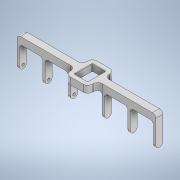
# Autodesk Inventor part: y arm connection
Saved by Autodesk Inventor 2021 (Build 250183000, 183)
## iProperties
Created: 2021-06-24
Part Number: y arm connection
Material: Generic
Document SubType Name: Modeling
Designer: josep
Density: 1 g/cm^3
Appearance: Default
Author: josep
Autodesk Inventor part; units mm, degrees
ref_plane "YZ Plane" through (0, 0, 0) normal (1, 0, 0) x (0, 1, 0)
ref_plane "XZ Plane" through (0, 0, 0) normal (0, 1, 0) x (-1, 0, 0)
ref_plane "XY Plane" through (0, 0, 0) normal (0, 0, 1) x (1, 0, 0)
sketch "Sketch1" plane through (0, 0, 0) normal (1, 0, 0) x (0, 1, 0)
  line L0 (0, 0) -> (0, -19)
  line L1 (0, 0) -> (0, 19)
  line L2 (0, 19) -> (-50, 19)
  line L3 (-50, 19) -> (-50, 29)
  line L4 (-50, 29) -> (0, 29)
  line L5 (0, 29) -> (0, 19)
  line L6 (0, -19) -> (-50, -19)
  line L7 (-50, -19) -> (-50, -29)
  line L8 (-50, -29) -> (0, -29)
  line L9 (0, -29) -> (0, -19)
  dimension "d0" = 19
  dimension "d1" = 19
  dimension "d2" = 50
  dimension "d3" = 10
  dimension "d4" = 50
  dimension "d5" = 10
  constraints: 20 end point, 4 perpendicular, 2 horizontal, 2 parallel, 2 vertical
  measures "d0" distance of L0.start L0.end
  measures "d1" distance of L0.start L1.end
  measures "d2" distance of L1.end L2.end
  measures "d3" distance of L2.end L3.end
  measures "d4" distance of L8.end L7.end
  measures "d5" distance of L7.end L6.end
extrude "Extrusion1" add sketch "Sketch1" along normal blind 347
sketch "Sketch2" plane through (0, 0, -19) normal (0, 1, 0) x (1, 0, 0)
  line L0 (-41.2158, -120.6879) -> (285.948, -120.6879)
  line L1 (285.948, -120.6879) -> (285.948, 128.9897)
  line L2 (285.948, 128.9897) -> (-41.2158, 128.9897)
  line L3 (-41.2158, 128.9897) -> (-41.2158, -120.6879)
  line L4 (-65.3226, -208.5055) -> (414.2306, -208.5055)
  line L5 (414.2306, -208.5055) -> (414.2306, 175.4814)
  line L6 (414.2306, 175.4814) -> (-65.3226, 175.4814)
  line L7 (-65.3226, 175.4814) -> (-65.3226, -208.5055)
  point P0 (0, -19)
  constraints: 16 end point, 4 parallel, 2 horizontal, 2 perpendicular
extrude "Extrusion2" cut sketch "Sketch2" against normal blind 25 contours L3 L2 L1 L0 | L7 L6 L5 L4
sketch "Sketch3" plane through (347, 0, 0) normal (1, 0, 0) x (0, 0, -1)
  line L0 (-29, -25) -> (-29, -50) projected
  line L1 (-29, -38.3566) -> (-26.5, -38.3566)
  line L2 (-26.5, -38.3566) -> (-25.5, -38.3566)
  line L3 (-29, -25) -> (-19, -25) projected
  line L4 (-25.5, -25) -> (-25.5, -50)
  line L5 (-29, -50) -> (-19, -50) projected
  line L6 (-29, -25) -> (-25.5, -25)
  line L7 (-25.5, -25) -> (-25.5, -50)
  line L8 (-25.5, -50) -> (-29, -50)
  line L9 (-29, -50) -> (-29, -25)
  line L10 (19, -50) -> (29, -50) projected
  line L11 (29, -25) -> (25.5, -25)
  line L12 (25.5, -25) -> (25.5, -50)
  line L13 (25.5, -50) -> (29, -50)
  line L14 (29, -50) -> (29, -25)
  point P0 (0, 0)
  dimension "d10" = 2.5
  dimension "d11" = 1
  dimension "d12" = 3.5
  constraints: 22 end point, 5 point on line, 4 parallel, 3 horizontal, 2 perpendicular, 1 vertical
  measures "d10" distance of L1.start L1.end
  measures "d11" distance of L1.end L2.end
  measures "d12" distance of L13.end L12.end
extrude "Extrusion3" cut sketch "Sketch3" against normal blind 373
sketch "Sketch4" plane through (0, -25, -19) normal (0, 1, 0) x (1, 0, 0)
  line L0 (0, -38) -> (347, -38) projected
  line L1 (277.7024, -38) -> (249.7024, -38)
  line L2 (249.7024, -38) -> (249.7024, 0)
  line L3 (347, 0) -> (0, 0) projected
  line L4 (277.7024, -38) -> (277.7024, 0)
  line L5 (277.7024, 0) -> (287.7024, 0)
  line L6 (287.7024, -36.5) -> (287.7024, -38)
  line L7 (229.7024, -11.5) -> (205.0573, -11.5)
  line L8 (297.7024, -11.5) -> (336.2476, -11.5)
  line L9 (336.2476, -11.5) -> (336.2476, -26.5)
  line L10 (336.2476, -26.5) -> (297.7024, -26.5)
  arc A0 (297.7024, -26.5) -> (287.7024, -36.5) centre (297.7024, -36.5) ccw
  line L11 (287.7024, 0) -> (287.7024, -1.5)
  arc A1 (287.7024, -1.5) -> (297.7024, -11.5) centre (297.7024, -1.5) ccw
  line L12 (287.7024, -38) -> (277.7024, -38)
  line L13 (249.7024, 0) -> (239.7024, 0)
  line L14 (239.7024, 0) -> (239.7024, -1.5)
  line L15 (239.7024, -36.5) -> (239.7024, -38)
  line L16 (229.7024, -26.5) -> (205.0573, -26.5)
  line L17 (205.0573, -26.5) -> (205.0573, -11.5)
  arc A2 (229.7024, -11.5) -> (239.7024, -1.5) centre (229.7024, -1.5) ccw
  arc A3 (239.7024, -36.5) -> (229.7024, -26.5) centre (229.7024, -36.5) ccw
  line L18 (249.7024, -38) -> (239.7024, -38)
  point P0 (0, -19)
  point P1 (239.7024, -19)
  point P2 (334.5589, -26.5)
  dimension "d15" = 28
  dimension "d16" = 10
  dimension "d19" = 15
  dimension "d20" = 10
  dimension "d21" = 10
  dimension "d22" = 10
  dimension "d23" = 10
  constraints: 34 end point, 17 point on line, 8 perpendicular, 8 point on circle, 8 tangent, 4 centre point, 2 collinear, 1 equal radius
  measures "d15" distance of L1.start L1.end
  measures "d16" distance of L4.end L5.end
  measures "d19" distance of L8.end L9.end
  measures "d20" radius of A0
  measures "d21" radius of A1
  measures "d22" distance of L2.end L13.end
  measures "d23" radius of A2
extrude "Extrusion4" add sketch "Sketch4" against normal blind 25 contours L15 A3 L16 L17 L7 A2 L14 L3 L2 L0 | L4 L3 L11 A1 L8 L9 L10 A0 L6 L0
sketch "Sketch5" plane through (0, -25, -19) normal (0, 1, 0) x (1, 0, 0)
  line L0 (249.7024, -38) -> (277.7024, -38) projected
  line L1 (277.7024, -38) -> (277.7024, -48)
  line L2 (277.7024, -48) -> (249.7024, -48)
  line L3 (347, -44.5) -> (0, -44.5) projected
  line L4 (287.7024, -38) -> (347, -38) projected
  line L5 (287.7024, -38) -> (287.7024, 0)
  arc A0 (277.7024, -48) -> (287.7024, -38) centre (277.7024, -38) ccw
  arc A1 (239.7024, -36.5) -> (229.7024, -26.5) centre (229.7024, -36.5) ccw projected
  line L6 (239.7024, 0) -> (239.7024, -38)
  arc A2 (239.7024, -38) -> (249.7024, -48) centre (249.7024, -38) ccw
  line L7 (249.7024, 0) -> (277.7024, 0) projected
  line L8 (277.7024, 0) -> (277.7024, 10)
  line L9 (277.7024, 10) -> (249.7024, 10)
  arc A3 (287.7024, 0) -> (277.7024, 10) centre (277.7024, 0) ccw
  arc A4 (249.7024, 10) -> (239.7024, 0) centre (249.7024, 0) ccw
  line L10 (277.7024, -38) -> (249.7024, -38)
  line L11 (249.7024, -38) -> (249.7024, 0)
  line L12 (249.7024, 0) -> (277.7024, 0)
  line L13 (277.7024, 0) -> (277.7024, -38)
  point P0 (0, -19)
  dimension "d26" = 10
  dimension "d27" = 10
  dimension "d28" = 10
  dimension "d29" = 10
  dimension "d30" = 10
  constraints: 20 end point, 9 tangent, 8 point on circle, 4 centre point, 4 point on line, 3 parallel, 3 perpendicular, 3 vertical, 1 equal radius, 1 horizontal
  measures "d26" distance of L0.end L1.end
  measures "d27" radius of A0
  measures "d28" radius of A2
  measures "d29" distance of L7.end L8.end
  measures "d30" radius of A3
extrude "Extrusion5" add sketch "Sketch5" against normal blind 25 contours L0 L1 L3 A2 L6 A4 L9 L8 L7 L11 | L13 L8 A3 L5 A0 L3 L1 | L3 A0 L1 | L1 L2 A2 L3
sketch "Sketch6" plane through (0, -25, -19) normal (0, 1, 0) x (1, 0, 0)
  arc A0 (287.7024, -1.5) -> (297.7024, -11.5) centre (297.7024, -1.5) ccw projected
  arc A1 (297.7024, -26.5) -> (287.7024, -36.5) centre (297.7024, -36.5) ccw projected
  line L0 (277.7024, -48) -> (249.7024, -48) projected
  line L1 (249.7024, -48) -> (277.7024, -48)
  arc A2 (277.7024, -48) -> (287.7024, -38) centre (277.7024, -38) ccw
  line L2 (249.7024, 10) -> (277.7024, 10) projected
  line L3 (277.7024, 10) -> (249.7024, 10)
  line L4 (239.7024, -36.5) -> (239.7024, -38) projected
  arc A3 (287.7024, 0) -> (277.7024, 10) centre (277.7024, 0) ccw
  arc A4 (249.7024, 10) -> (239.7024, 0) centre (249.7024, 0) ccw
  arc A5 (239.7024, -38) -> (249.7024, -48) centre (249.7024, -38) ccw
  line L5 (395.5953, -66.3707) -> (-113.6205, -66.3707)
  line L6 (-113.6205, -66.3707) -> (-113.6205, 72.1294)
  line L7 (-113.6205, 72.1294) -> (395.5953, 72.1294)
  line L8 (395.5953, 72.1294) -> (395.5953, -66.3707)
  line L9 (287.7024, -38) -> (349.7072, -27.7131)
  line L10 (349.7072, -27.7131) -> (348.1864, -4.5628)
  line L11 (348.1864, -4.5628) -> (318.7048, -5.5764)
  line L12 (318.7048, -5.5764) -> (293.2276, -4.5628)
  line L13 (347, 0) -> (287.7024, 0) projected
  line L14 (287.7024, 0) -> (293.2276, -4.5628)
  line L15 (0, -38) -> (239.7024, -38) projected
  line L16 (239.7024, -38) -> (183.3233, -27.7131)
  line L17 (183.3233, -27.7131) -> (188.9622, -13.5346)
  line L18 (239.7024, 0) -> (239.7024, -1.5) projected
  line L19 (188.9622, -13.5346) -> (239.7024, 0)
  point P0 (0, -19)
  point P1 (256.6196, -48)
  point P2 (272.9773, -48)
  point P3 (272.9773, 10)
  point P4 (258.3118, 10)
  dimension "d33" = 10
  dimension "d34" = 10
  constraints: 28 end point, 8 point on circle, 8 point on line, 4 centre point, 4 tangent, 2 equal radius, 2 parallel, 1 horizontal, 1 perpendicular
  measures "d33" radius of A2
  measures "d34" radius of A3
extrude "Extrusion6" cut sketch "Sketch6" against normal blind 113.5
sketch "Sketch7" plane through (336.2476, -25, 7.5) normal (1, 0, 0) x (0, 0, -1)
  line L0 (26.5, -25) -> (-11.5, -25) projected
  line L1 (15, 0) -> (15, -25) projected
  line L2 (-0.0488, -25) -> (15, -25)
  line L3 (15, -25) -> (15, 0)
  line L4 (15, 0) -> (-0.0488, 0)
  line L5 (-0.0488, 0) -> (-0.0488, -25)
  point P0 (7.5, 25)
  constraints: 8 end point, 2 parallel, 1 horizontal, 1 perpendicular, 1 point on line
extrude "Extrusion7" add sketch "Sketch7" along normal blind 320
sketch "Sketch8" plane through (205.0573, -50, 7.5) normal (0, -1, 0) x (1, 0, 0)
  arc A0 (34.6451, -25) -> (24.6451, -15) centre (24.6451, -25) ccw projected
  line L0 (24.6451, 0) -> (0, 0) projected
  line L1 (24.6451, -15) -> (19.6451, -15)
  line L2 (19.6451, -15) -> (19.6451, 0)
  line L3 (19.6451, 0) -> (24.6451, 0)
  line L4 (24.6451, 0) -> (24.6451, -15)
  point P0 (-205.0573, -7.5)
  dimension "d39" = 5
  constraints: 8 end point, 2 parallel, 1 horizontal, 1 perpendicular, 1 point on line
  measures "d39" distance of L2.end L3.end
extrude "Extrusion8" add sketch "Sketch8" along normal blind 50
sketch "Sketch9" plane through (224.7024, -50, -7.5) normal (-1, 0, 0) x (0, 0, 1)
  line L0 (0, -50) -> (15, -50) projected
  line L1 (7.5, -50) -> (7.5, -42.5)
  circle A0 centre (7.5, -42.5) radius 7.5
  line L2 (0, 0) -> (0, -50) projected
  line L3 (0, -42.5) -> (15, -42.5)
  line L4 (15, -42.5) -> (15, -50)
  line L5 (15, -50) -> (0, -50)
  line L6 (0, -50) -> (0, -42.5)
  point P0 (7.5, 50)
  point P1 (15, -42.5)
  dimension "d42" = 7.5
  constraints: 10 end point, 2 parallel, 2 point on circle, 1 centre point, 1 coincident, 1 horizontal, 1 midpoint, 1 perpendicular, 1 point on line, 1 vertical
  measures "d42" distance of L1.start L1.end
extrude "Extrusion9" cut sketch "Sketch9" against normal blind 50 contours L2 A0 L0 | A0 L4 L0
sketch "Sketch10" plane through (205.0573, -25, -7.5) normal (-1, 0, 0) x (0, 0, 1)
  line L0 (0, 0) -> (0, -25) projected
  line L1 (15, -25) -> (0, -25) projected
  line L2 (0, 0) -> (15, 0)
  line L3 (15, 0) -> (15, -25)
  line L4 (15, -25) -> (0, -25)
  line L5 (0, -25) -> (0, 0)
  point P0 (7.5, 25)
  constraints: 8 end point, 2 parallel, 1 horizontal, 1 perpendicular
extrude "Extrusion10" add sketch "Sketch10" along normal blind 318.75
sketch "Sketch11" plane through (224.7024, -50, -7.5) normal (0, -1, 0) x (1, 0, 0)
  line L0 (0, 0) -> (0, 15) projected
  line L1 (0, 7.5) -> (-50, 7.5)
  line L2 (0, 0) -> (-338.3951, 0) projected
  line L3 (0, 15) -> (-338.3951, 15) projected
  line L4 (-50, 0) -> (-55, 0)
  line L5 (-55, 0) -> (-55, 15)
  line L6 (-55, 15) -> (-50, 15)
  line L7 (-50, 15) -> (-50, 0)
  line L8 (-55, 7.5) -> (-105, 7.5)
  line L9 (-105, 0) -> (-110, 0)
  line L10 (-110, 0) -> (-110, 15)
  line L11 (-110, 15) -> (-105, 15)
  line L12 (-105, 15) -> (-105, 0)
  point P0 (-224.7024, 7.5)
  point P1 (-55, 0)
  point P2 (-110, 0)
  dimension "d47" = 50
  dimension "d48" = 5
  dimension "d49" = 50
  dimension "d50" = 5
  constraints: 20 end point, 4 horizontal, 4 parallel, 4 point on line, 2 midpoint, 2 perpendicular
  measures "d47" distance of L1.start L1.end
  measures "d48" distance of L5.end L6.end
  measures "d49" distance of L8.start L8.end
  measures "d50" distance of L10.end L11.end
extrude "Extrusion11" add sketch "Sketch11" along normal blind 50 contours L2 L5 L3 L7 | L2 L10 L3 L12
sketch "Sketch12" plane through (-113.6927, -50, -7.5) normal (0, -1, 0) x (1, 0, 0)
  line L0 (228.3951, 15) -> (228.3951, 0) projected
  line L1 (228.3951, 15) -> (-4838.5654, 15)
  line L2 (-4838.5654, 15) -> (-4838.5654, -3335.2499)
  line L3 (-4838.5654, -3335.2499) -> (228.3951, -3335.2499)
  line L4 (228.3951, -3335.2499) -> (228.3951, 15)
  point P0 (113.6927, 7.5)
  constraints: 8 end point, 2 parallel, 1 horizontal, 1 perpendicular
extrude "Extrusion12" cut sketch "Sketch12" against normal blind 50
sketch "Sketch13" plane through (114.7024, -100, -7.5) normal (-1, 0, 0) x (0, 0, 1)
  line L0 (15, 0) -> (0, 0) projected
  line L1 (7.5, 0) -> (7.5, 7.5)
  circle A0 centre (7.5, 7.5) radius 7.5
  line L2 (0, 50) -> (0, 7.5) projected
  line L3 (0, 7.5) -> (15, 7.5)
  line L4 (15, 7.5) -> (15, 0)
  line L5 (15, 0) -> (0, 0)
  line L6 (0, 0) -> (0, 7.5)
  point P0 (7.5, 100)
  point P1 (15, 7.5)
  dimension "d55" = 7.5
  constraints: 10 end point, 2 parallel, 1 centre point, 1 coincident, 1 horizontal, 1 midpoint, 1 perpendicular, 1 point on circle, 1 vertical
  measures "d55" distance of L1.start L1.end
sketch "Sketch14" plane through (277.7024, -25, -19) normal (-1, 0, 0) x (0, 0, 1)
  line L0 (38, -25) -> (0, -25) projected
  line L1 (38, 0) -> (0, 0)
  line L2 (0, 0) -> (0, -25)
  line L3 (0, -25) -> (38, -25)
  line L4 (38, -25) -> (38, 0)
  point P0 (19, 25)
  constraints: 8 end point, 2 parallel, 1 horizontal, 1 perpendicular
extrude "Extrusion13" add sketch "Sketch14" along normal blind 14
extrude "Extrusion14" cut sketch "Sketch13" against normal blind 183 contours L0 A0 L4 | L0 L6 A0
sketch "Sketch15" plane through (229.7024, -50, 7.5) normal (1, 0, 0) x (0, 0, -1)
  arc A0 (0, -42.5) -> (15, -42.5) centre (7.5, -42.5) ccw projected
  circle A1 centre (7.5, -42.5) radius 2.925
  point P0 (7.5, 50)
  dimension "d60" = 5.85
  constraints: 1 centre point, 1 coincident
  measures "d60" diameter of A1
extrude "Extrusion15" cut sketch "Sketch15" against normal blind 3.5
sketch "Sketch16" plane through (174.7024, -50, 7.5) normal (1, 0, 0) x (0, 0, -1)
  circle A0 centre (7.5, -42.5) radius 2.925
  point P0 (7.5, 50)
  dimension "d63" = 5.85
  constraints: 1 centre point
  measures "d63" diameter of A0
extrude "Extrusion16" cut sketch "Sketch16" against normal blind 3.5
sketch "Sketch17" plane through (119.7024, -50, 7.5) normal (1, 0, 0) x (0, 0, -1)
  arc A0 (0, -42.5) -> (15, -42.5) centre (7.5, -42.5) ccw projected
  circle A1 centre (7.5, -42.5) radius 2.925
  point P0 (7.5, 50)
  dimension "d66" = 5.85
  constraints: 1 centre point, 1 coincident
  measures "d66" diameter of A1
extrude "Extrusion17" cut sketch "Sketch17" against normal blind 3.5
sketch "Sketch18" plane through (263.7024, -25, -19) normal (-1, 0, 0) x (0, 0, 1)
  line L0 (-90.6404, 73.0269) -> (201.3127, 73.0269)
  line L1 (201.3127, 73.0269) -> (201.3127, -129.1917)
  line L2 (201.3127, -129.1917) -> (-90.6404, -129.1917)
  line L3 (-90.6404, -129.1917) -> (-90.6404, 73.0269)
  point P0 (19, 25)
  constraints: 8 end point, 2 parallel, 1 horizontal, 1 perpendicular
extrude "Extrusion18" cut sketch "Sketch18" against normal blind 599
mirror "Mirror1" about plane through (263.7024, -53.0824, 36.3362) normal (1, 0, 0)
sketch "Sketch19" plane through (0, -25, -19) normal (0, 1, 0) x (1, 0, 0)
  line L0 (36.6559, 37.945) -> (601.2573, 37.945)
  line L1 (601.2573, 37.945) -> (601.2573, -148.0607)
  line L2 (601.2573, -148.0607) -> (36.6559, -148.0607)
  line L3 (36.6559, -148.0607) -> (36.6559, 37.945)
  point P0 (0, -19)
  constraints: 8 end point, 2 parallel, 1 horizontal, 1 perpendicular
extrude "Extrusion19" cut sketch "Sketch19" against normal blind 10
fillet "Fillet1" radius 7 12 edges at (412.7024, -35, 0) (114.7024, -35, 0) (119.7024, -50, 0) (407.7024, -50, 0) (352.7024, -50, 0) (224.7024, -50, 0) (169.7024, -50, 0) (174.7024, -50, 0) (229.7024, -50, 0) (302.7024, -50, 0) (357.7024, -50, 0) (297.7024, -50, 0)
fillet "Fillet2" radius 1 12 edges at (263.7024, -35, 19) (249.7024, -35, 0) (277.7024, -35, 0) (263.7024, -35, -19) (263.7024, -50, -19) (277.7024, -50, 0) (263.7024, -50, 19) (249.7024, -50, 0) (249.7024, -42.5, 19) (277.7024, -42.5, 19) (277.7024, -42.5, -19) (249.7024, -42.5, -19)
body "Solid1"
